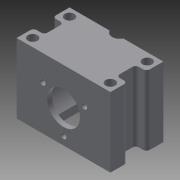
# Autodesk Inventor part: EncoderSupportInside
Saved by Autodesk Inventor 2014 SP1 (Build 180222100, 222)
## iProperties
Created: 2015-03-28
Part Number: EncoderSupportInside
Material: Generic
Document SubType Name: Modeling
Designer: david
Density: 1 g/cm^3
Appearance: Default
EncoderSupportInside_Length: 33,000 mm
EncoderSupportInside_Width: 58,500 mm
EncoderSupportInside_Height: 46,500 mm
EncoderSupportInside_Thickness: 6,000 mm
EncoderSupportInside_Front_Thickness: 3,000 mm
EncoderSupportInside_Hollow_Margin: 2,500 mm
EncoderSupportInside_Hollow_WidthDistanceToCenter: 22,500 mm
EncoderSupport_Fillet_Size: 2,000 mm
EncoderSupport_PlasticShrinkingMargin: 0,500 mm
EncoderSupport_CoilSpringHole_Diameter: 6,000 mm
EncoderSupport_FixingHole_Diameter: 3,000 mm
EncoderSupport_FixingnHole_Margin: 5,000 mm
EncoderSupportInside_FasteningHole_WidthDistanceToCenter: 24,250 mm
Author: david
Autodesk Inventor part; units mm, degrees
ref_plane "YZ Plane" through (0, 0, 0) normal (1, 0, 0) x (0, 1, 0)
ref_plane "XZ Plane" through (0, 0, 0) normal (0, 1, 0) x (-1, 0, 0)
ref_plane "XY Plane" through (0, 0, 0) normal (0, 0, 1) x (1, 0, 0)
sketch "FrontSketch" plane through (0, 0, 0) normal (0, 0, 1) x (1, 0, 0)
  line L0 (0, 0) -> (0, 22.8261) construction
  line L1 (0, 0) -> (24.783, 0) construction
  circle A0 centre (0, 0) radius 10.25
  circle A1 centre (0, 0) radius 20.25 construction
  line L2 (-29.25, 23.25) -> (29.25, 23.25)
  line L3 (29.25, 23.25) -> (29.25, -20.25)
  line L4 (29.25, -20.25) -> (-29.25, -20.25)
  line L5 (-29.25, -20.25) -> (-29.25, 23.25)
  line L6 (0, 0) -> (-39.7334, 0) construction
  circle A2 centre (0, 0) radius 15 construction
  circle A3 centre (0, -15) radius 1.75
  line L7 (0, 0) -> (0, -25.6264) construction
  circle A4 centre (12.9904, 7.5) radius 1.75
  circle A5 centre (-12.9904, 7.5) radius 1.75
  point P0 (0, 20.25)
  point P1 (-20.25, 0)
  dimension "d25" = 30
  dimension "d21" = 20.5
  dimension "d22" = 40.5
  dimension "d23" = 9
  dimension "d24" = 3
  dimension "d26" = 3.5
  dimension "d29" = 360
  constraints: 16 end point, 5 centre point, 5 coincident, 4 perpendicular, 3 point on line, 2 parallel, 2 point on circle, 1 horizontal, 1 tangent, 1 vertical alignment, 10 other
  measures "d21" diameter of A0
  measures "d22" diameter of A1
  measures "d23" distance from line of L5 A1.start
  measures "d24" distance from line of L2 A1.end
  measures "d26" diameter of A3
extrude "Front" add sketch "FrontSketch" along normal blind 3
sketch "FerruleSketch" plane through (0, 0, 0) normal (0, 0, -1) x (-1, 0, 0)
  circle A0 centre (0, 0) radius 10.25 projected
  line L0 (29.25, 23.25) -> (-29.25, 23.25) projected
  line L1 (-29.25, 23.25) -> (-29.25, -20.25) projected
  line L2 (-29.25, -20.25) -> (29.25, -20.25) projected
  line L3 (29.25, -20.25) -> (29.25, 23.25) projected
  circle A1 centre (0, 0) radius 20.25
  dimension "d33" = 40.5
  constraints: 1 centre point, 1 coincident
  measures "d33" diameter of A1
extrude "Ferrule" add sketch "FerruleSketch" along normal blind 30 contours L3 L2 L1 L0
sketch "Sketch7" plane through (0, 0, -30) normal (0, 0, -1) x (-1, 0, 0)
  line L0 (-29.25, -20.25) -> (29.25, -20.25) projected
  circle A0 centre (0, 0) radius 20.25 projected
  line L1 (-29.25, -20.25) -> (29.25, -20.25) projected
  line L2 (29.25, -20.25) -> (29.25, 23.25) projected
  line L3 (13.3229, -15.25) -> (13.3229, -20.25)
  line L4 (-13.3229, -15.25) -> (-13.3229, -20.25)
  line L5 (0, 0) -> (0, -25.3199) construction
  point P0 (0, -20.25)
  dimension "d37" = 5
  constraints: 6 end point, 3 parallel, 2 point on circle, 2 point on line, 1 other
  measures "d37" distance of L3.start L3.end
extrude "Extrusion8" cut sketch "Sketch7" against normal up to surface (30 mm away) contours L4 A0 L0 | A0 L3 L0
sketch "CableHoleSketch" plane through (-29.25, 23.25, 3) normal (0, 1, 0) x (1, 0, 0)
  line L0 (0, 33) -> (58.5, 33) projected
  line L1 (29.25, 3) -> (29.25, 34.9321) construction
  circle A0 centre (29.25, 35) radius 4.75
  line L2 (49.5, 3) -> (9, 3) projected
  line L3 (24.9416, 33) -> (33.5584, 33)
  point P0 (15.9271, 3)
  point P1 (42.5729, 3)
  dimension "d40" = 32
  dimension "d41" = 9.5
  constraints: 4 end point, 3 point on line, 2 point on circle, 1 centre point, 1 perpendicular
  measures "d40" distance from line of L2 A0.centre
  measures "d41" diameter of A0
extrude "CableHole" cut sketch "CableHoleSketch" against normal up to next contours L0 A0 picked at (29.25, 32.0833)
sketch "FasteningHoleSketch" plane through (-29.25, 23.25, 3) normal (0, 1, 0) x (1, 0, 0)
  arc A0 (24.9416, 33) -> (33.5584, 33) centre (29.25, 35) ccw projected
  line L0 (33.5584, 33) -> (58.5, 33) projected
  circle A1 centre (5, 5) radius 1.5
  line L1 (29.25, 3) -> (29.25, 35) construction
  line L2 (58.5, 0) -> (0, 0) projected
  line L3 (58.5, 0) -> (58.5, 33) projected
  line L4 (-10.6096, 16.5) -> (55.9901, 16.5) construction
  circle A2 centre (5, 28) radius 1.5
  line L5 (29.25, 30) -> (29.25, -2) construction
  circle A3 centre (53.5, 5) radius 1.5
  circle A4 centre (53.5, 28) radius 1.5
  dimension "d44" = 3
  dimension "d45" = 5
  dimension "d53" = 16.5
  constraints: 6 end point, 5 symmetric about line, 4 centre point, 2 perpendicular, 4 other
  measures "d44" diameter of A1
  measures "d45" horizontal distance of L2.end A1.centre
  measures "d53" distance between parallel lines of L2 L4
extrude "FasteningHole" cut sketch "FasteningHoleSketch" against normal blind 41.5
sketch "CoilSpringHoleSketch" plane through (-29.25, 23.25, 3) normal (0, 1, 0) x (1, 0, 0)
  circle A0 centre (53.5, 5) radius 1.5 projected
  circle A1 centre (5, 5) radius 1.5 projected
  circle A2 centre (5, 28) radius 1.5 projected
  circle A3 centre (53.5, 28) radius 1.5 projected
  arc A4 (24.9416, 33) -> (33.5584, 33) centre (29.25, 35) ccw projected
  line L0 (58.5, 0) -> (0, 0) projected
  line L1 (33.5584, 33) -> (58.5, 33) projected
  circle A5 centre (5, 28) radius 3
  line L2 (29.25, 3) -> (29.25, 35) construction
  line L3 (-9.4478, 16.5) -> (72.8784, 16.5) construction
  circle A6 centre (53.5, 28) radius 3
  circle A7 centre (5, 5) radius 3
  circle A8 centre (53.5, 5) radius 3
  dimension "d54" = 6
  dimension "d55" = 16.5
  constraints: 4 centre point, 4 end point, 3 symmetric about line, 2 perpendicular, 1 coincident, 3 other
  measures "d54" diameter of A5
  measures "d55" distance between parallel lines of L3 L0
extrude "CoilSpringHole" cut sketch "CoilSpringHoleSketch" against normal blind 13
sketch "HollowSketch" plane through (-29.25, 23.25, 3) normal (0, 1, 0) x (1, 0, 0)
  circle A0 centre (5, 28) radius 3 projected
  arc A1 (24.9416, 33) -> (33.5584, 33) centre (29.25, 35) ccw projected
  line L0 (0, 33) -> (0, 0) projected
  line L1 (58.5, 0) -> (0, 0) projected
  line L2 (0, 22.5) -> (6.75, 22.5)
  line L3 (6.75, 22.5) -> (6.75, 10.5)
  line L4 (6.75, 10.5) -> (0, 10.5)
  line L5 (0, 10.5) -> (0, 22.5)
  line L6 (29.25, 35) -> (29.25, 3) construction
  line L7 (58.5, 22.5) -> (51.75, 22.5)
  line L8 (51.75, 22.5) -> (51.75, 10.5)
  line L9 (51.75, 10.5) -> (58.5, 10.5)
  line L10 (58.5, 10.5) -> (58.5, 22.5)
  line L11 (-4.7611, 16.5) -> (67.4575, 16.5) construction
  line L12 (9.25, 35.7853) -> (9.25, -4.0496) construction
  dimension "d58" = 16.5
  dimension "d59" = 20
  dimension "d60" = 2.5
  dimension "d61" = 2.5
  constraints: 22 end point, 4 symmetric about line, 3 parallel, 3 perpendicular, 1 horizontal, 1 point on line, 1 other
  measures "d58" distance between parallel lines of L1 L11
  measures "d59" distance between parallel lines of L6 L12
  measures "d60" distance between parallel lines of L12 L3
  measures "d61" distance edge to line of A0 L2
extrude "Hollow" cut sketch "HollowSketch" against normal up to next contours L2 L3 L4 L0 | L10 L9 L8 L7
fillet "Fillet2" radius 2 8 edges at (-22.5, 1.5, -7.5) (-29.25, 1.5, -7.5) (-22.5, 1.5, -19.5) (-29.25, 1.5, -19.5) (29.25, 1.5, -19.5) (29.25, 1.5, -7.5) (22.5, 1.5, -19.5) (22.5, 1.5, -7.5)
equation "\"d25\" = 2 * Encoder_FasteningHole_DistanceToCenter"
equation "\"d21\" = Encoder_Bearing_Diameter + EncoderSupport_PlasticShrinkingMargin"
equation "\"d22\" = Encoder_Body_Diameter + EncoderSupport_PlasticShrinkingMargin"
equation "\"d23\" = EncoderSupportInside_SideThickness"
equation "\"d24\" = EncoderSupportInside_TopThickness"
equation "\"d26\" = Encoder_FasteningHole_Diameter + EncoderSupport_PlasticShrinkingMargin"
equation "\"d33\" = Encoder_Body_Diameter + EncoderSupport_PlasticShrinkingMargin"
equation "\"d40\" = Encoder_CableBase_DistanceToTop"
equation "\"d41\" = Encoder_CableBase_Diameter + EncoderSupport_PlasticShrinkingMargin"
equation "\"d44\" = EncoderSupport_FixingHole_Diameter"
equation "\"d45\" = EncoderSupport_FixingnHole_Margin"
equation "\"d53\" = 0.5 * EncoderSupportInside_Length"
equation "\"d54\" = EncoderSupport_CoilSpringHole_Diameter"
equation "\"d55\" = 0.5 * EncoderSupportInside_Length"
equation "\"d58\" = 0.5 * EncoderSupportInside_Length"
equation "\"d59\" = 0.5 * Encoder_Body_Diameter"
equation "\"d60\" = EncoderSupportInside_Hollow_Margin"
equation "\"d61\" = EncoderSupportInside_Hollow_Margin"
equation "\"d65\" = EncoderSupport_Fillet_Size"
equation "\"EncoderSupportInside_Thickness\" = 6"
equation "\"EncoderSupportInside_Length\" = EncoderSupportInside_Front_Thickness + d34"
equation "\"EncoderSupportInside_Width\" = EncoderSupport_PlasticShrinkingMargin + Encoder_Body_Diameter + 2 * EncoderSupportInside_SideThickness"
equation "\"EncoderSupportInside_Height\" = EncoderSupport_PlasticShrinkingMargin + Encoder_Body_Diameter + EncoderSupportInside_Thickness"
equation "\"EncoderSupport_FixingHole_Diameter\" = 3"
equation "\"EncoderSupport_FixingnHole_Margin\" = 5"
equation "\"EncoderSupportInside_SideThickness\" = EncoderSupportInside_Thickness + EncoderSupport_FixingHole_Diameter"
equation "\"EncoderSupport_CoilSpringHole_Diameter\" = 6"
equation "\"EncoderSupportInside_TopThickness\" = 3"
equation "\"EncoderSupportInside_Hollow_Margin\" = 2.5"
equation "\"EncoderSupport_Fillet_Size\" = 2"
equation "\"EncoderSupport_PlasticShrinkingMargin\" = 0.5"
equation "\"Encoder_FasteningHole_DistanceToCenter\" = 15"
equation "\"Encoder_Bearing_Diameter\" = 20"
equation "\"Encoder_Body_Diameter\" = 40"
equation "\"Encoder_FasteningHole_Diameter\" = 3"
equation "\"Encoder_CableBase_DistanceToTop\" = 32"
equation "\"Encoder_CableBase_Diameter\" = 9"
equation "\"EncoderSupportInside_Front_Thickness\" = 3"
equation "\"d34\" = 30"
body "Solid2"
